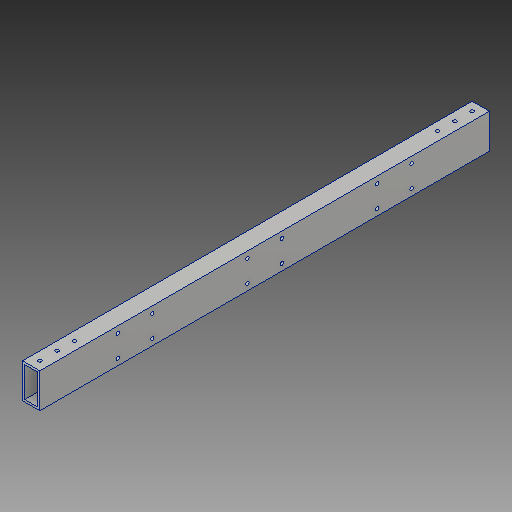
# Autodesk Inventor part: 26 1x2
Saved by Autodesk Inventor 2018 (Build 220112000, 112)
## iProperties
Created: 2018-09-23
Part Number: 26 1x2
Material: Aluminum 6061
Document SubType Name: Modeling
Designer: maste
Density: 2.7 g/cm^3
Appearance: Aluminum - Flat
Author: maste
Autodesk Inventor part; units mm, degrees
ref_plane "YZ Plane" through (0, 0, 0) normal (1, 0, 0) x (0, 1, 0)
ref_plane "XZ Plane" through (0, 0, 0) normal (0, 1, 0) x (-1, 0, 0)
ref_plane "XY Plane" through (0, 0, 0) normal (0, 0, 1) x (1, 0, 0)
sketch "Sketch1" plane through (0, 0, 0) normal (0, 0, 1) x (1, 0, 0)
  line L0 (0, 0) -> (25.4, 0)
  line L1 (25.4, 0) -> (25.4, 50.8)
  line L2 (25.4, 50.8) -> (0, 50.8)
  line L3 (0, 50.8) -> (0, 0)
  line L4 (3.175, 3.175) -> (22.225, 3.175)
  line L5 (22.225, 3.175) -> (22.225, 47.625)
  line L6 (22.225, 47.625) -> (3.175, 47.625)
  line L7 (3.175, 47.625) -> (3.175, 3.175)
  dimension "d0" = 25.4
  dimension "d1" = 50.8
  dimension "d2" = 3.175
  dimension "d3" = 3.175
  dimension "d4" = 3.175
  dimension "d5" = 3.175
  constraints: 16 end point, 4 parallel, 2 horizontal, 2 perpendicular
  measures "d0" distance of L2.end L1.end
  measures "d1" distance of L1.end L0.end
  measures "d2" distance between parallel lines of L2 L6
  measures "d3" distance between parallel lines of L0 L4
  measures "d4" distance between parallel lines of L7 L3
  measures "d5" distance between parallel lines of L5 L1
extrude "Extrusion1" add sketch "Sketch1" along normal blind 660.4
sketch "Sketch2" plane through (0, 50.8, 0) normal (0, 1, 0) x (1, 0, 0)
  line L0 (25.4, 0) -> (0, 0) projected
  line L1 (12.7, 0) -> (12.7, -660.4)
  line L2 (0, -660.4) -> (25.4, -660.4) projected
  line L3 (12.7, -660.4) -> (12.7, -647.7)
  line L4 (12.7, -647.7) -> (12.7, -622.3)
  line L5 (12.7, -622.3) -> (12.7, -596.9)
  circle A0 centre (12.7, -647.7) radius 2.54
  circle A1 centre (12.7, -622.3) radius 2.54
  circle A2 centre (12.7, -596.9) radius 2.54
  line L6 (12.7, 0) -> (12.7, -12.7)
  line L7 (12.7, -12.7) -> (12.7, -38.1)
  line L8 (12.7, -38.1) -> (12.7, -63.5)
  circle A3 centre (12.7, -63.5) radius 2.54
  circle A4 centre (12.7, -38.1) radius 2.54
  circle A5 centre (12.7, -12.7) radius 2.54
  dimension "d8" = 12.7
  dimension "d9" = 25.4
  dimension "d10" = 25.4
  dimension "d11" = 5.08
  dimension "d12" = 12.7
  dimension "d13" = 25.4
  dimension "d14" = 25.4
  constraints: 14 end point, 6 centre point, 6 coincident, 6 point on line, 2 midpoint
  measures "d8" distance of L1.end L3.end
  measures "d9" distance of L3.end L4.end
  measures "d10" distance of L4.end L5.end
  measures "d11" diameter of A0
  measures "d12" distance of L1.start L6.end
  measures "d13" distance of L6.end L7.end
  measures "d14" distance of L7.end L8.end
extrude "Extrusion2" cut sketch "Sketch2" against normal blind 660.4
sketch "Sketch3" plane through (25.4, 0, 0) normal (1, 0, 0) x (0, 0, -1)
  line L0 (0, 50.8) -> (-660.4, 50.8) projected
  line L1 (0, 50.8) -> (-114.3, 50.8)
  line L2 (-114.3, 50.8) -> (-165.1, 50.8)
  line L3 (-114.3, 50.8) -> (-114.3, 41.275)
  line L4 (-165.1, 50.8) -> (-165.1, 41.275)
  circle A0 centre (-165.1, 41.275) radius 2.54
  circle A1 centre (-114.3, 41.275) radius 2.54
  line L5 (-165.1, 0) -> (-165.1, 9.525)
  line L6 (0, 0) -> (-660.4, 0) projected
  line L7 (-114.3, 0) -> (-114.3, 9.525)
  circle A2 centre (-165.1, 9.525) radius 2.54
  circle A3 centre (-114.3, 9.525) radius 2.54
  dimension "d17" = 114.3
  dimension "d18" = 50.8
  dimension "d19" = 9.525
  dimension "d20" = 5.08
  dimension "d21" = 9.525
  constraints: 12 end point, 4 centre point, 4 coincident, 4 vertical, 3 point on line
  measures "d17" distance of L0.start L1.end
  measures "d18" distance of L1.end L2.end
  measures "d19" distance of L1.end L3.end
  measures "d20" diameter of A0
  measures "d21" distance of L5.start L5.end
extrude "Extrusion3" cut sketch "Sketch3" against normal blind 660.4
sketch "Sketch4" plane through (25.4, 0, 0) normal (1, 0, 0) x (0, 0, -1)
  circle A0 centre (-165.1, 41.275) radius 2.54 projected
  line L0 (-165.1, 41.275) -> (-304.8, 41.275)
  line L1 (-304.8, 41.275) -> (-355.6, 41.275)
  line L2 (-355.6, 41.275) -> (-355.6, 9.525)
  line L3 (-355.6, 9.525) -> (-304.8, 9.525)
  circle A1 centre (-304.8, 41.275) radius 2.54
  circle A2 centre (-355.6, 41.275) radius 2.54
  circle A3 centre (-355.6, 9.525) radius 2.54
  circle A4 centre (-304.8, 9.525) radius 2.54
  point P0 (0, 0)
  dimension "d24" = 139.7
  dimension "d25" = 50.8
  constraints: 8 end point, 4 centre point, 4 coincident, 2 perpendicular, 1 horizontal, 1 point on line
  measures "d24" distance of L0.start L0.end
  measures "d25" distance of L0.end L1.end
extrude "Extrusion4" cut sketch "Sketch4" against normal blind 660.4 contours A4 | A3 L3 L2 | L2 L3 A3 | A2 L2 L1 | L1 L2 A2 | A1 L1 L0 | L0 L1 A1
sketch "Sketch5" plane through (25.4, 0, 0) normal (1, 0, 0) x (0, 0, -1)
  circle A0 centre (-355.6, 41.275) radius 2.54 projected
  line L0 (-355.6, 41.275) -> (-495.3, 41.275)
  line L1 (-495.3, 41.275) -> (-546.1, 41.275)
  line L2 (-546.1, 41.275) -> (-546.1, 9.525)
  line L3 (-546.1, 9.525) -> (-495.3, 9.525)
  circle A1 centre (-495.3, 41.275) radius 2.54
  circle A2 centre (-546.1, 41.275) radius 2.54
  circle A3 centre (-546.1, 9.525) radius 2.54
  circle A4 centre (-495.3, 9.525) radius 2.54
  point P0 (0, 0)
  dimension "d28" = 139.7
  dimension "d29" = 50.8
  constraints: 8 end point, 4 centre point, 4 coincident, 2 perpendicular, 1 horizontal, 1 point on line
  measures "d28" distance of L0.start L0.end
  measures "d29" distance of L0.end L1.end
extrude "Extrusion5" cut sketch "Sketch5" against normal blind 660.4 contours A4 | A3 L3 L2 | L2 L3 A3 | A2 L2 L1 | L1 L2 A2 | A1 L1 L0 | L0 L1 A1
body "Solid1"
